Autodesk Fusion 360 part; units mm, degrees
note: some values were not read from the file. Set by a fixed rule: which sketch regions a step uses.
(part 11 of 20)
sketch "スケッチ2 (2)" plane through (0, 0, 8) normal (0, 0, 1) x (-1, 0, 0)
  circle A0 centre (-7.0711, -7.0711) radius 1.7
  circle A1 centre (7.0711, 7.0711) radius 1.7
  circle A2 centre (0, 10) radius 1.7
  circle A3 centre (0, -10) radius 1.7
  circle A4 centre (-10, 0) radius 1.7
  circle A5 centre (10, 0) radius 1.7
  circle A6 centre (-7.0711, 7.0711) radius 1.7
  circle A7 centre (7.0711, -7.0711) radius 1.7
  arc A8 (-13.5924, 2.0756) -> (-13.727, 0.7957) centre (0, 0) ccw
  line L0 (-13.727, 0.7957) -> (-14.4979, 0.8404)
  line L1 (-14.4979, 0.8404) -> (-14.4985, 0.8405)
  spline S0 degree 5 poles (-14.4985, 0.8405) (-14.4986, 0.8405) (-14.4987, 0.8405) (-14.499, 0.8405) (-14.4993, 0.8405) (-14.4999, 0.8405) (-14.5005, 0.8406) (-14.5012, 0.8406) (-14.502, 0.8406) (-14.5028, 0.8406) (-14.5037, 0.8407) (-14.5048, 0.8407) (-14.5058, 0.8407) (-14.507, 0.8407) (-14.5082, 0.8408) (-14.5096, 0.8408) (-14.5109, 0.8408) (-14.5124, 0.8408) (-14.5139, 0.8409) (-14.5155, 0.8409) (-14.5172, 0.8409) (-14.519, 0.8409) (-14.5208, 0.8409) (-14.5226, 0.8409) (-14.5246, 0.8409) (-14.5266, 0.8409) (-14.5287, 0.8409) (-14.5309, 0.8409) (-14.5331, 0.8408) (-14.5354, 0.8408) (-14.5377, 0.8408) (-14.5401, 0.8407) (-14.5426, 0.8407) (-14.5452, 0.8406) (-14.5478, 0.8406) (-14.5504, 0.8405) (-14.5532, 0.8404) (-14.556, 0.8403) (-14.5588, 0.8402) (-14.5617, 0.8401) (-14.5647, 0.84) (-14.5677, 0.8399) (-14.5708, 0.8398) (-14.574, 0.8396) (-14.5772, 0.8395) (-14.5805, 0.8393) (-14.5838, 0.8392) (-14.5872, 0.839) (-14.5906, 0.8388) (-14.5941, 0.8386) (-14.5977, 0.8384) (-14.6013, 0.8382) (-14.605, 0.838) (-14.6087, 0.8377) (-14.6124, 0.8375) (-14.6163, 0.8372) (-14.6202, 0.8369) (-14.6241, 0.8366) (-14.6281, 0.8363) (-14.6321, 0.836) (-14.6362, 0.8357) (-14.6404, 0.8354) (-14.6446, 0.835) (-14.6488, 0.8347) (-14.6531, 0.8343) (-14.6574, 0.8339) (-14.6618, 0.8335) (-14.6663, 0.8331) (-14.6708, 0.8326) (-14.6753, 0.8322) (-14.6799, 0.8317) (-14.6846, 0.8313) (-14.6893, 0.8308) (-14.694, 0.8303) (-14.6988, 0.8298) (-14.7036, 0.8292) (-14.7085, 0.8287) (-14.7134, 0.8281) (-14.7184, 0.8275) (-14.7234, 0.8269) (-14.7285, 0.8263) (-14.7336, 0.8257) (-14.7387, 0.8251) (-14.7439, 0.8244) (-14.7492, 0.8237) (-14.7545, 0.8231) (-14.7598, 0.8224) (-14.7652, 0.8216) (-14.7706, 0.8209) (-14.7761, 0.8201) (-14.7816, 0.8194) (-14.7871, 0.8186) (-14.7927, 0.8178) (-14.7983, 0.817) (-14.804, 0.8161) (-14.8097, 0.8153) (-14.8155, 0.8144) (-14.8213, 0.8135) (-14.8271, 0.8126) (-14.833, 0.8117) (-14.8389, 0.8107) (-14.8449, 0.8097) (-14.8509, 0.8088) (-14.8569, 0.8078) (-14.863, 0.8067) (-14.8691, 0.8057) (-14.8753, 0.8047) (-14.8814, 0.8036) (-14.8877, 0.8025) (-14.8939, 0.8014) (-14.9003, 0.8002) (-14.9066, 0.7991) (-14.913, 0.7979) (-14.9194, 0.7967) (-14.9259, 0.7955) (-14.9324, 0.7943) (-14.9389, 0.7931) (-14.9455, 0.7918) (-14.9521, 0.7905) (-14.9587, 0.7892) (-14.9654, 0.7879) (-14.9721, 0.7865) (-14.9788, 0.7852) (-14.9856, 0.7838) (-14.9924, 0.7824) (-14.9993, 0.781) (-15.0062, 0.7795) (-15.0131, 0.778) (-15.02, 0.7766) (-15.027, 0.775) (-15.0341, 0.7735) (-15.0411, 0.772) (-15.0482, 0.7704) (-15.0553, 0.7688) (-15.0625, 0.7672) (-15.0697, 0.7656) (-15.0769, 0.7639) (-15.0841, 0.7622) (-15.0914, 0.7605) (-15.0987, 0.7588) (-15.1061, 0.7571) (-15.1135, 0.7553) (-15.1209, 0.7535) (-15.1283, 0.7517) (-15.1358, 0.7499) (-15.1433, 0.7481) (-15.1508, 0.7462) (-15.1584, 0.7443) (-15.166, 0.7424) (-15.1736, 0.7405) (-15.1813, 0.7385) (-15.1889, 0.7365) (-15.1967, 0.7345) (-15.2044, 0.7325) (-15.2122, 0.7305) (-15.22, 0.7284) (-15.2278, 0.7263) (-15.2357, 0.7242) (-15.2436, 0.7221) (-15.2515, 0.7199) (-15.2594, 0.7177) (-15.2674, 0.7155) (-15.2754, 0.7133) (-15.2834, 0.7111) (-15.2915, 0.7088) (-15.2996, 0.7065) (-15.3077, 0.7042) (-15.3158, 0.7018) (-15.324, 0.6995) (-15.3322, 0.6971) (-15.3404, 0.6947) (-15.3487, 0.6923) (-15.3569, 0.6898) (-15.3652, 0.6873) (-15.3736, 0.6848) (-15.3819, 0.6823) (-15.3903, 0.6797) (-15.3987, 0.6772) (-15.4071, 0.6746) (-15.4156, 0.672) (-15.4241, 0.6693) (-15.4326, 0.6667) (-15.4411, 0.664) (-15.4497, 0.6613) (-15.4582, 0.6585) (-15.4668, 0.6558) (-15.4755, 0.653) (-15.4841, 0.6502) (-15.4928, 0.6473) (-15.5015, 0.6445) (-15.5102, 0.6416) (-15.519, 0.6387) (-15.5278, 0.6358) (-15.5365, 0.6328) (-15.5454, 0.6298) (-15.5542, 0.6268) (-15.5631, 0.6238) (-15.572, 0.6207) (-15.5809, 0.6177) (-15.5898, 0.6146) (-15.5988, 0.6114) (-15.6077, 0.6083) (-15.6167, 0.6051) (-15.6258, 0.6019) (-15.6348, 0.5987) (-15.6439, 0.5955) (-15.653, 0.5922) (-15.6621, 0.5889) (-15.6712, 0.5856) (-15.6803, 0.5822) (-15.6895, 0.5789) (-15.6987, 0.5755) (-15.7079, 0.572) (-15.7172, 0.5686) (-15.7264, 0.5651) (-15.7357, 0.5616) (-15.745, 0.5581) (-15.7543, 0.5546) (-15.7636, 0.551) (-15.773, 0.5474) (-15.7824, 0.5438) (-15.7918, 0.5401) (-15.8012, 0.5365) (-15.8106, 0.5328) (-15.8201, 0.529) (-15.8295, 0.5253) (-15.839, 0.5215) (-15.8486, 0.5177) (-15.8581, 0.5139) (-15.8676, 0.5101) (-15.8772, 0.5062) (-15.8868, 0.5023) (-15.8964, 0.4984) (-15.906, 0.4944) (-15.9157, 0.4904) (-15.9253, 0.4864) (-15.935, 0.4824) (-15.9447, 0.4784) (-15.9544, 0.4743) (-15.9641, 0.4702) (-15.9739, 0.466) (-15.9817, 0.4627) (-15.9876, 0.4602) (-15.9915, 0.4585) (-15.9935, 0.4577) knots 0 0 0 0 0 0 0.00416667 0.00833333 0.0125 0.01666667 0.02083333 0.025 0.02916667 0.03333333 0.0375 0.04166667 0.04583333 0.05 0.05416667 0.05833333 0.0625 0.06666667 0.07083333 0.075 0.07916667 0.08333333 0.0875 0.09166667 0.09583333 0.1 0.10416667 0.10833333 0.1125 0.11666667 0.12083333 0.125 0.12916667 0.13333333 0.1375 0.14166667 0.14583333 0.15 0.15416667 0.15833333 0.1625 0.16666667 0.17083333 0.175 0.17916667 0.18333333 0.1875 0.19166667 0.19583333 0.2 0.20416667 0.20833333 0.2125 0.21666667 0.22083333 0.225 0.22916667 0.23333333 0.2375 0.24166667 0.24583333 0.25 0.25416667 0.25833333 0.2625 0.26666667 0.27083333 0.275 0.27916667 0.28333333 0.2875 0.29166667 0.29583333 0.3 0.30416667 0.30833333 0.3125 0.31666667 0.32083333 0.325 0.32916667 0.33333333 0.3375 0.34166667 0.34583333 0.35 0.35416667 0.35833333 0.3625 0.36666667 0.37083333 0.375 0.37916667 0.38333333 0.3875 0.39166667 0.39583333 0.4 0.40416667 0.40833333 0.4125 0.41666667 0.42083333 0.425 0.42916667 0.43333333 0.4375 0.44166667 0.44583333 0.45 0.45416667 0.45833333 0.4625 0.46666667 0.47083333 0.475 0.47916667 0.48333333 0.4875 0.49166667 0.49583333 0.5 0.50416667 0.50833333 0.5125 0.51666667 0.52083333 0.525 0.52916667 0.53333333 0.5375 0.54166667 0.54583333 0.55 0.55416667 0.55833333 0.5625 0.56666667 0.57083333 0.575 0.57916667 0.58333333 0.5875 0.59166667 0.59583333 0.6 0.60416667 0.60833333 0.6125 0.61666667 0.62083333 0.625 0.62916667 0.63333333 0.6375 0.64166667 0.64583333 0.65 0.65416667 0.65833333 0.6625 0.66666667 0.67083333 0.675 0.67916667 0.68333333 0.6875 0.69166667 0.69583333 0.7 0.70416667 0.70833333 0.7125 0.71666667 0.72083333 0.725 0.72916667 0.73333333 0.7375 0.74166667 0.74583333 0.75 0.75416667 0.75833333 0.7625 0.76666667 0.77083333 0.775 0.77916667 0.78333333 0.7875 0.79166667 0.79583333 0.8 0.80416667 0.80833333 0.8125 0.81666667 0.82083333 0.825 0.82916667 0.83333333 0.8375 0.84166667 0.84583333 0.85 0.85416667 0.85833333 0.8625 0.86666667 0.87083333 0.875 0.87916667 0.88333333 0.8875 0.89166667 0.89583333 0.9 0.90416667 0.90833333 0.9125 0.91666667 0.92083333 0.925 0.92916667 0.93333333 0.9375 0.94166667 0.94583333 0.95 0.95416667 0.95833333 0.9625 0.96666667 0.97083333 0.975 0.97916667 0.98333333 0.9875 0.99166667 0.99583333 1 1 1 1 1 1
  arc A9 (-15.9935, 0.4577) -> (-15.9935, -0.4577) centre (0, 0) ccw
  spline S1 degree 5 poles (-15.9935, -0.4577) (-15.9915, -0.4585) (-15.9876, -0.4602) (-15.9817, -0.4627) (-15.9739, -0.466) (-15.9641, -0.4702) (-15.9544, -0.4743) (-15.9447, -0.4784) (-15.935, -0.4824) (-15.9253, -0.4864) (-15.9157, -0.4904) (-15.906, -0.4944) (-15.8964, -0.4984) (-15.8868, -0.5023) (-15.8772, -0.5062) (-15.8676, -0.5101) (-15.8581, -0.5139) (-15.8486, -0.5177) (-15.839, -0.5215) (-15.8295, -0.5253) (-15.8201, -0.529) (-15.8106, -0.5328) (-15.8012, -0.5365) (-15.7918, -0.5401) (-15.7824, -0.5438) (-15.773, -0.5474) (-15.7636, -0.551) (-15.7543, -0.5546) (-15.745, -0.5581) (-15.7357, -0.5616) (-15.7264, -0.5651) (-15.7172, -0.5686) (-15.7079, -0.572) (-15.6987, -0.5755) (-15.6895, -0.5789) (-15.6803, -0.5822) (-15.6712, -0.5856) (-15.6621, -0.5889) (-15.653, -0.5922) (-15.6439, -0.5955) (-15.6348, -0.5987) (-15.6258, -0.6019) (-15.6167, -0.6051) (-15.6077, -0.6083) (-15.5988, -0.6114) (-15.5898, -0.6146) (-15.5809, -0.6177) (-15.572, -0.6207) (-15.5631, -0.6238) (-15.5542, -0.6268) (-15.5454, -0.6298) (-15.5365, -0.6328) (-15.5278, -0.6358) (-15.519, -0.6387) (-15.5102, -0.6416) (-15.5015, -0.6445) (-15.4928, -0.6473) (-15.4841, -0.6502) (-15.4755, -0.653) (-15.4668, -0.6558) (-15.4582, -0.6585) (-15.4497, -0.6613) (-15.4411, -0.664) (-15.4326, -0.6667) (-15.4241, -0.6693) (-15.4156, -0.672) (-15.4071, -0.6746) (-15.3987, -0.6772) (-15.3903, -0.6797) (-15.3819, -0.6823) (-15.3736, -0.6848) (-15.3652, -0.6873) (-15.3569, -0.6898) (-15.3487, -0.6923) (-15.3404, -0.6947) (-15.3322, -0.6971) (-15.324, -0.6995) (-15.3158, -0.7018) (-15.3077, -0.7042) (-15.2996, -0.7065) (-15.2915, -0.7088) (-15.2834, -0.7111) (-15.2754, -0.7133) (-15.2674, -0.7155) (-15.2594, -0.7177) (-15.2515, -0.7199) (-15.2436, -0.7221) (-15.2357, -0.7242) (-15.2278, -0.7263) (-15.22, -0.7284) (-15.2122, -0.7305) (-15.2044, -0.7325) (-15.1967, -0.7345) (-15.1889, -0.7365) (-15.1813, -0.7385) (-15.1736, -0.7405) (-15.166, -0.7424) (-15.1584, -0.7443) (-15.1508, -0.7462) (-15.1433, -0.7481) (-15.1358, -0.7499) (-15.1283, -0.7517) (-15.1209, -0.7535) (-15.1135, -0.7553) (-15.1061, -0.7571) (-15.0987, -0.7588) (-15.0914, -0.7605) (-15.0841, -0.7622) (-15.0769, -0.7639) (-15.0697, -0.7656) (-15.0625, -0.7672) (-15.0553, -0.7688) (-15.0482, -0.7704) (-15.0411, -0.772) (-15.0341, -0.7735) (-15.027, -0.775) (-15.02, -0.7766) (-15.0131, -0.778) (-15.0062, -0.7795) (-14.9993, -0.781) (-14.9924, -0.7824) (-14.9856, -0.7838) (-14.9788, -0.7852) (-14.9721, -0.7865) (-14.9654, -0.7879) (-14.9587, -0.7892) (-14.9521, -0.7905) (-14.9455, -0.7918) (-14.9389, -0.7931) (-14.9324, -0.7943) (-14.9259, -0.7955) (-14.9194, -0.7967) (-14.913, -0.7979) (-14.9066, -0.7991) (-14.9003, -0.8002) (-14.8939, -0.8014) (-14.8877, -0.8025) (-14.8814, -0.8036) (-14.8753, -0.8047) (-14.8691, -0.8057) (-14.863, -0.8067) (-14.8569, -0.8078) (-14.8509, -0.8088) (-14.8449, -0.8097) (-14.8389, -0.8107) (-14.833, -0.8117) (-14.8271, -0.8126) (-14.8213, -0.8135) (-14.8155, -0.8144) (-14.8097, -0.8153) (-14.804, -0.8161) (-14.7983, -0.817) (-14.7927, -0.8178) (-14.7871, -0.8186) (-14.7816, -0.8194) (-14.7761, -0.8201) (-14.7706, -0.8209) (-14.7652, -0.8216) (-14.7598, -0.8224) (-14.7545, -0.8231) (-14.7492, -0.8237) (-14.7439, -0.8244) (-14.7387, -0.8251) (-14.7336, -0.8257) (-14.7285, -0.8263) (-14.7234, -0.8269) (-14.7184, -0.8275) (-14.7134, -0.8281) (-14.7085, -0.8287) (-14.7036, -0.8292) (-14.6988, -0.8298) (-14.694, -0.8303) (-14.6893, -0.8308) (-14.6846, -0.8313) (-14.6799, -0.8317) (-14.6753, -0.8322) (-14.6708, -0.8326) (-14.6663, -0.8331) (-14.6618, -0.8335) (-14.6574, -0.8339) (-14.6531, -0.8343) (-14.6488, -0.8347) (-14.6446, -0.835) (-14.6404, -0.8354) (-14.6362, -0.8357) (-14.6321, -0.836) (-14.6281, -0.8363) (-14.6241, -0.8366) (-14.6202, -0.8369) (-14.6163, -0.8372) (-14.6124, -0.8375) (-14.6087, -0.8377) (-14.605, -0.838) (-14.6013, -0.8382) (-14.5977, -0.8384) (-14.5941, -0.8386) (-14.5906, -0.8388) (-14.5872, -0.839) (-14.5838, -0.8392) (-14.5805, -0.8393) (-14.5772, -0.8395) (-14.574, -0.8396) (-14.5708, -0.8398) (-14.5677, -0.8399) (-14.5647, -0.84) (-14.5617, -0.8401) (-14.5588, -0.8402) (-14.556, -0.8403) (-14.5532, -0.8404) (-14.5504, -0.8405) (-14.5478, -0.8406) (-14.5452, -0.8406) (-14.5426, -0.8407) (-14.5401, -0.8407) (-14.5377, -0.8408) (-14.5354, -0.8408) (-14.5331, -0.8408) (-14.5309, -0.8409) (-14.5287, -0.8409) (-14.5266, -0.8409) (-14.5246, -0.8409) (-14.5226, -0.8409) (-14.5208, -0.8409) (-14.519, -0.8409) (-14.5172, -0.8409) (-14.5155, -0.8409) (-14.5139, -0.8409) (-14.5124, -0.8408) (-14.5109, -0.8408) (-14.5096, -0.8408) (-14.5082, -0.8408) (-14.507, -0.8407) (-14.5058, -0.8407) (-14.5048, -0.8407) (-14.5037, -0.8407) (-14.5028, -0.8406) (-14.502, -0.8406) (-14.5012, -0.8406) (-14.5005, -0.8406) (-14.4999, -0.8405) (-14.4993, -0.8405) (-14.499, -0.8405) (-14.4987, -0.8405) (-14.4986, -0.8405) (-14.4985, -0.8405) knots -1 -1 -1 -1 -1 -1 -0.99583333 -0.99166667 -0.9875 -0.98333333 -0.97916667 -0.975 -0.97083333 -0.96666667 -0.9625 -0.95833333 -0.95416667 -0.95 -0.94583333 -0.94166667 -0.9375 -0.93333333 -0.92916667 -0.925 -0.92083333 -0.91666667 -0.9125 -0.90833333 -0.90416667 -0.9 -0.89583333 -0.89166667 -0.8875 -0.88333333 -0.87916667 -0.875 -0.87083333 -0.86666667 -0.8625 -0.85833333 -0.85416667 -0.85 -0.84583333 -0.84166667 -0.8375 -0.83333333 -0.82916667 -0.825 -0.82083333 -0.81666667 -0.8125 -0.80833333 -0.80416667 -0.8 -0.79583333 -0.79166667 -0.7875 -0.78333333 -0.77916667 -0.775 -0.77083333 -0.76666667 -0.7625 -0.75833333 -0.75416667 -0.75 -0.74583333 -0.74166667 -0.7375 -0.73333333 -0.72916667 -0.725 -0.72083333 -0.71666667 -0.7125 -0.70833333 -0.70416667 -0.7 -0.69583333 -0.69166667 -0.6875 -0.68333333 -0.67916667 -0.675 -0.67083333 -0.66666667 -0.6625 -0.65833333 -0.65416667 -0.65 -0.64583333 -0.64166667 -0.6375 -0.63333333 -0.62916667 -0.625 -0.62083333 -0.61666667 -0.6125 -0.60833333 -0.60416667 -0.6 -0.59583333 -0.59166667 -0.5875 -0.58333333 -0.57916667 -0.575 -0.57083333 -0.56666667 -0.5625 -0.55833333 -0.55416667 -0.55 -0.54583333 -0.54166667 -0.5375 -0.53333333 -0.52916667 -0.525 -0.52083333 -0.51666667 -0.5125 -0.50833333 -0.50416667 -0.5 -0.49583333 -0.49166667 -0.4875 -0.48333333 -0.47916667 -0.475 -0.47083333 -0.46666667 -0.4625 -0.45833333 -0.45416667 -0.45 -0.44583333 -0.44166667 -0.4375 -0.43333333 -0.42916667 -0.425 -0.42083333 -0.41666667 -0.4125 -0.40833333 -0.40416667 -0.4 -0.39583333 -0.39166667 -0.3875 -0.38333333 -0.37916667 -0.375 -0.37083333 -0.36666667 -0.3625 -0.35833333 -0.35416667 -0.35 -0.34583333 -0.34166667 -0.3375 -0.33333333 -0.32916667 -0.325 -0.32083333 -0.31666667 -0.3125 -0.30833333 -0.30416667 -0.3 -0.29583333 -0.29166667 -0.2875 -0.28333333 -0.27916667 -0.275 -0.27083333 -0.26666667 -0.2625 -0.25833333 -0.25416667 -0.25 -0.24583333 -0.24166667 -0.2375 -0.23333333 -0.22916667 -0.225 -0.22083333 -0.21666667 -0.2125 -0.20833333 -0.20416667 -0.2 -0.19583333 -0.19166667 -0.1875 -0.18333333 -0.17916667 -0.175 -0.17083333 -0.16666667 -0.1625 -0.15833333 -0.15416667 -0.15 -0.14583333 -0.14166667 -0.1375 -0.13333333 -0.12916667 -0.125 -0.12083333 -0.11666667 -0.1125 -0.10833333 -0.10416667 -0.1 -0.09583333 -0.09166667 -0.0875 -0.08333333 -0.07916667 -0.075 -0.07083333 -0.06666667 -0.0625 -0.05833333 -0.05416667 -0.05 -0.04583333 -0.04166667 -0.0375 -0.03333333 -0.02916667 -0.025 -0.02083333 -0.01666667 -0.0125 -0.00833333 -0.00416667 0 0 0 0 0 0
  line L2 (-14.4985, -0.8405) -> (-14.4979, -0.8404)
  line L3 (-14.4979, -0.8404) -> (-13.727, -0.7957)
  arc A10 (-13.727, -0.7957) -> (-13.5924, -2.0756) centre (0, 0) ccw
  line L4 (-13.5924, -2.0756) -> (-14.3558, -2.1922)
  line L5 (-14.3558, -2.1922) -> (-14.3564, -2.1923)
  spline S2 degree 5 poles (-14.3564, -2.1923) (-14.3565, -2.1923) (-14.3566, -2.1923) (-14.3569, -2.1924) (-14.3572, -2.1924) (-14.3578, -2.1925) (-14.3584, -2.1926) (-14.3591, -2.1928) (-14.3598, -2.1929) (-14.3607, -2.193) (-14.3616, -2.1932) (-14.3626, -2.1934) (-14.3637, -2.1936) (-14.3648, -2.1938) (-14.366, -2.194) (-14.3673, -2.1943) (-14.3687, -2.1945) (-14.3701, -2.1948) (-14.3716, -2.1951) (-14.3732, -2.1954) (-14.3748, -2.1958) (-14.3765, -2.1961) (-14.3783, -2.1965) (-14.3801, -2.1969) (-14.382, -2.1973) (-14.384, -2.1977) (-14.386, -2.1982) (-14.3882, -2.1986) (-14.3903, -2.1991) (-14.3925, -2.1996) (-14.3948, -2.2002) (-14.3972, -2.2007) (-14.3996, -2.2013) (-14.4021, -2.2018) (-14.4046, -2.2025) (-14.4072, -2.2031) (-14.4099, -2.2037) (-14.4126, -2.2044) (-14.4154, -2.2051) (-14.4182, -2.2058) (-14.4211, -2.2065) (-14.424, -2.2072) (-14.427, -2.208) (-14.4301, -2.2088) (-14.4332, -2.2096) (-14.4364, -2.2104) (-14.4396, -2.2113) (-14.4429, -2.2122) (-14.4462, -2.2131) (-14.4496, -2.214) (-14.453, -2.2149) (-14.4565, -2.2159) (-14.46, -2.2169) (-14.4636, -2.2179) (-14.4673, -2.2189) (-14.4709, -2.22) (-14.4747, -2.2211) (-14.4785, -2.2222) (-14.4823, -2.2233) (-14.4862, -2.2244) (-14.4901, -2.2256) (-14.4941, -2.2268) (-14.4981, -2.228) (-14.5022, -2.2292) (-14.5063, -2.2305) (-14.5105, -2.2318) (-14.5147, -2.2331) (-14.519, -2.2344) (-14.5233, -2.2358) (-14.5277, -2.2372) (-14.5321, -2.2386) (-14.5365, -2.24) (-14.541, -2.2414) (-14.5455, -2.2429) (-14.5501, -2.2444) (-14.5547, -2.2459) (-14.5594, -2.2475) (-14.5641, -2.2491) (-14.5688, -2.2507) (-14.5736, -2.2523) (-14.5784, -2.2539) (-14.5833, -2.2556) (-14.5882, -2.2573) (-14.5932, -2.259) (-14.5981, -2.2608) (-14.6032, -2.2626) (-14.6082, -2.2644) (-14.6133, -2.2662) (-14.6185, -2.268) (-14.6237, -2.2699) (-14.6289, -2.2718) (-14.6342, -2.2737) (-14.6395, -2.2757) (-14.6448, -2.2776) (-14.6502, -2.2796) (-14.6556, -2.2817) (-14.661, -2.2837) (-14.6665, -2.2858) (-14.672, -2.2879) (-14.6776, -2.29) (-14.6832, -2.2922) (-14.6888, -2.2944) (-14.6945, -2.2966) (-14.7002, -2.2988) (-14.7059, -2.3011) (-14.7117, -2.3034) (-14.7175, -2.3057) (-14.7233, -2.308) (-14.7292, -2.3104) (-14.7351, -2.3128) (-14.741, -2.3152) (-14.747, -2.3176) (-14.753, -2.3201) (-14.759, -2.3226) (-14.7651, -2.3251) (-14.7712, -2.3277) (-14.7773, -2.3302) (-14.7835, -2.3328) (-14.7897, -2.3355) (-14.7959, -2.3381) (-14.8022, -2.3408) (-14.8084, -2.3435) (-14.8148, -2.3463) (-14.8211, -2.349) (-14.8275, -2.3518) (-14.8339, -2.3546) (-14.8403, -2.3575) (-14.8468, -2.3604) (-14.8533, -2.3633) (-14.8598, -2.3662) (-14.8663, -2.3691) (-14.8729, -2.3721) (-14.8795, -2.3751) (-14.8862, -2.3782) (-14.8928, -2.3812) (-14.8995, -2.3843) (-14.9062, -2.3874) (-14.913, -2.3906) (-14.9198, -2.3938) (-14.9266, -2.397) (-14.9334, -2.4002) (-14.9402, -2.4034) (-14.9471, -2.4067) (-14.954, -2.41) (-14.9609, -2.4134) (-14.9679, -2.4167) (-14.9749, -2.4201) (-14.9819, -2.4236) (-14.9889, -2.427) (-14.996, -2.4305) (-15.0031, -2.434) (-15.0102, -2.4375) (-15.0173, -2.4411) (-15.0245, -2.4447) (-15.0316, -2.4483) (-15.0388, -2.4519) (-15.0461, -2.4556) (-15.0533, -2.4593) (-15.0606, -2.463) (-15.0679, -2.4668) (-15.0752, -2.4706) (-15.0825, -2.4744) (-15.0899, -2.4782) (-15.0973, -2.4821) (-15.1047, -2.486) (-15.1121, -2.4899) (-15.1196, -2.4939) (-15.1271, -2.4978) (-15.1346, -2.5018) (-15.1421, -2.5059) (-15.1496, -2.5099) (-15.1572, -2.514) (-15.1648, -2.5182) (-15.1724, -2.5223) (-15.18, -2.5265) (-15.1876, -2.5307) (-15.1953, -2.5349) (-15.203, -2.5392) (-15.2107, -2.5435) (-15.2184, -2.5478) (-15.2262, -2.5522) (-15.2339, -2.5565) (-15.2417, -2.5609) (-15.2495, -2.5654) (-15.2574, -2.5698) (-15.2652, -2.5743) (-15.2731, -2.5788) (-15.2809, -2.5834) (-15.2888, -2.588) (-15.2968, -2.5926) (-15.3047, -2.5972) (-15.3126, -2.6019) (-15.3206, -2.6065) (-15.3286, -2.6113) (-15.3366, -2.616) (-15.3446, -2.6208) (-15.3527, -2.6256) (-15.3607, -2.6304) (-15.3688, -2.6353) (-15.3769, -2.6402) (-15.385, -2.6451) (-15.3931, -2.65) (-15.4013, -2.655) (-15.4094, -2.66) (-15.4176, -2.665) (-15.4258, -2.6701) (-15.434, -2.6752) (-15.4422, -2.6803) (-15.4505, -2.6855) (-15.4587, -2.6906) (-15.467, -2.6958) (-15.4753, -2.7011) (-15.4836, -2.7063) (-15.4919, -2.7116) (-15.5002, -2.7169) (-15.5086, -2.7223) (-15.517, -2.7277) (-15.5253, -2.7331) (-15.5337, -2.7385) (-15.5421, -2.744) (-15.5505, -2.7494) (-15.559, -2.755) (-15.5674, -2.7605) (-15.5759, -2.7661) (-15.5844, -2.7717) (-15.5929, -2.7773) (-15.6014, -2.783) (-15.6099, -2.7887) (-15.6184, -2.7944) (-15.6269, -2.8002) (-15.6355, -2.8059) (-15.6441, -2.8117) (-15.6526, -2.8176) (-15.6612, -2.8234) (-15.6698, -2.8293) (-15.6785, -2.8353) (-15.6871, -2.8412) (-15.6957, -2.8472) (-15.7044, -2.8532) (-15.713, -2.8592) (-15.7217, -2.8653) (-15.7287, -2.8702) (-15.7339, -2.8738) (-15.7374, -2.8763) (-15.7391, -2.8775) knots 0 0 0 0 0 0 0.00416667 0.00833333 0.0125 0.01666667 0.02083333 0.025 0.02916667 0.03333333 0.0375 0.04166667 0.04583333 0.05 0.05416667 0.05833333 0.0625 0.06666667 0.07083333 0.075 0.07916667 0.08333333 0.0875 0.09166667 0.09583333 0.1 0.10416667 0.10833333 0.1125 0.11666667 0.12083333 0.125 0.12916667 0.13333333 0.1375 0.14166667 0.14583333 0.15 0.15416667 0.15833333 0.1625 0.16666667 0.17083333 0.175 0.17916667 0.18333333 0.1875 0.19166667 0.19583333 0.2 0.20416667 0.20833333 0.2125 0.21666667 0.22083333 0.225 0.22916667 0.23333333 0.2375 0.24166667 0.24583333 0.25 0.25416667 0.25833333 0.2625 0.26666667 0.27083333 0.275 0.27916667 0.28333333 0.2875 0.29166667 0.29583333 0.3 0.30416667 0.30833333 0.3125 0.31666667 0.32083333 0.325 0.32916667 0.33333333 0.3375 0.34166667 0.34583333 0.35 0.35416667 0.35833333 0.3625 0.36666667 0.37083333 0.375 0.37916667 0.38333333 0.3875 0.39166667 0.39583333 0.4 0.40416667 0.40833333 0.4125 0.41666667 0.42083333 0.425 0.42916667 0.43333333 0.4375 0.44166667 0.44583333 0.45 0.45416667 0.45833333 0.4625 0.46666667 0.47083333 0.475 0.47916667 0.48333333 0.4875 0.49166667 0.49583333 0.5 0.50416667 0.50833333 0.5125 0.51666667 0.52083333 0.525 0.52916667 0.53333333 0.5375 0.54166667 0.54583333 0.55 0.55416667 0.55833333 0.5625 0.56666667 0.57083333 0.575 0.57916667 0.58333333 0.5875 0.59166667 0.59583333 0.6 0.60416667 0.60833333 0.6125 0.61666667 0.62083333 0.625 0.62916667 0.63333333 0.6375 0.64166667 0.64583333 0.65 0.65416667 0.65833333 0.6625 0.66666667 0.67083333 0.675 0.67916667 0.68333333 0.6875 0.69166667 0.69583333 0.7 0.70416667 0.70833333 0.7125 0.71666667 0.72083333 0.725 0.72916667 0.73333333 0.7375 0.74166667 0.74583333 0.75 0.75416667 0.75833333 0.7625 0.76666667 0.77083333 0.775 0.77916667 0.78333333 0.7875 0.79166667 0.79583333 0.8 0.80416667 0.80833333 0.8125 0.81666667 0.82083333 0.825 0.82916667 0.83333333 0.8375 0.84166667 0.84583333 0.85 0.85416667 0.85833333 0.8625 0.86666667 0.87083333 0.875 0.87916667 0.88333333 0.8875 0.89166667 0.89583333 0.9 0.90416667 0.90833333 0.9125 0.91666667 0.92083333 0.925 0.92916667 0.93333333 0.9375 0.94166667 0.94583333 0.95 0.95416667 0.95833333 0.9625 0.96666667 0.97083333 0.975 0.97916667 0.98333333 0.9875 0.99166667 0.99583333 1 1 1 1 1 1
  arc A11 (-15.7391, -2.8775) -> (-15.5488, -3.7729) centre (0, 0) ccw
  spline S3 degree 5 poles (-15.5488, -3.7729) (-15.5467, -3.7733) (-15.5425, -3.7742) (-15.5363, -3.7754) (-15.5279, -3.777) (-15.5175, -3.779) (-15.5072, -3.781) (-15.4968, -3.783) (-15.4865, -3.7849) (-15.4762, -3.7869) (-15.4659, -3.7888) (-15.4556, -3.7907) (-15.4454, -3.7925) (-15.4352, -3.7944) (-15.425, -3.7962) (-15.4148, -3.798) (-15.4047, -3.7998) (-15.3946, -3.8015) (-15.3845, -3.8033) (-15.3744, -3.805) (-15.3644, -3.8067) (-15.3544, -3.8083) (-15.3444, -3.81) (-15.3344, -3.8116) (-15.3244, -3.8132) (-15.3145, -3.8148) (-15.3046, -3.8164) (-15.2947, -3.8179) (-15.2849, -3.8195) (-15.2751, -3.821) (-15.2653, -3.8225) (-15.2555, -3.8239) (-15.2457, -3.8254) (-15.236, -3.8268) (-15.2263, -3.8282) (-15.2166, -3.8296) (-15.207, -3.831) (-15.1974, -3.8323) (-15.1878, -3.8337) (-15.1782, -3.835) (-15.1687, -3.8363) (-15.1591, -3.8375) (-15.1497, -3.8388) (-15.1402, -3.84) (-15.1308, -3.8412) (-15.1214, -3.8424) (-15.112, -3.8436) (-15.1026, -3.8448) (-15.0933, -3.8459) (-15.084, -3.847) (-15.0747, -3.8481) (-15.0655, -3.8492) (-15.0563, -3.8503) (-15.0471, -3.8513) (-15.0379, -3.8523) (-15.0288, -3.8533) (-15.0197, -3.8543) (-15.0106, -3.8553) (-15.0015, -3.8562) (-14.9925, -3.8572) (-14.9835, -3.8581) (-14.9746, -3.859) (-14.9656, -3.8598) (-14.9567, -3.8607) (-14.9479, -3.8615) (-14.939, -3.8624) (-14.9302, -3.8632) (-14.9214, -3.8639) (-14.9127, -3.8647) (-14.9039, -3.8655) (-14.8952, -3.8662) (-14.8866, -3.8669) (-14.8779, -3.8676) (-14.8693, -3.8683) (-14.8608, -3.869) (-14.8522, -3.8696) (-14.8437, -3.8702) (-14.8352, -3.8708) (-14.8268, -3.8714) (-14.8184, -3.872) (-14.81, -3.8726) (-14.8016, -3.8731) (-14.7933, -3.8737) (-14.785, -3.8742) (-14.7768, -3.8747) (-14.7685, -3.8751) (-14.7603, -3.8756) (-14.7522, -3.8761) (-14.744, -3.8765) (-14.7359, -3.8769) (-14.7279, -3.8773) (-14.7199, -3.8777) (-14.7119, -3.878) (-14.7039, -3.8784) (-14.696, -3.8787) (-14.6881, -3.8791) (-14.6802, -3.8794) (-14.6724, -3.8797) (-14.6646, -3.8799) (-14.6568, -3.8802) (-14.6491, -3.8804) (-14.6414, -3.8807) (-14.6338, -3.8809) (-14.6261, -3.8811) (-14.6186, -3.8813) (-14.611, -3.8814) (-14.6035, -3.8816) (-14.596, -3.8817) (-14.5886, -3.8819) (-14.5812, -3.882) (-14.5738, -3.8821) (-14.5665, -3.8822) (-14.5592, -3.8823) (-14.5519, -3.8823) (-14.5447, -3.8824) (-14.5375, -3.8824) (-14.5304, -3.8824) (-14.5233, -3.8824) (-14.5162, -3.8824) (-14.5091, -3.8824) (-14.5021, -3.8824) (-14.4952, -3.8823) (-14.4883, -3.8823) (-14.4814, -3.8822) (-14.4745, -3.8821) (-14.4677, -3.882) (-14.461, -3.8819) (-14.4542, -3.8818) (-14.4476, -3.8817) (-14.4409, -3.8816) (-14.4343, -3.8814) (-14.4277, -3.8812) (-14.4212, -3.8811) (-14.4147, -3.8809) (-14.4083, -3.8807) (-14.4019, -3.8805) (-14.3955, -3.8803) (-14.3892, -3.88) (-14.3829, -3.8798) (-14.3767, -3.8796) (-14.3705, -3.8793) (-14.3643, -3.879) (-14.3582, -3.8788) (-14.3521, -3.8785) (-14.3461, -3.8782) (-14.3401, -3.8779) (-14.3342, -3.8776) (-14.3283, -3.8772) (-14.3224, -3.8769) (-14.3166, -3.8766) (-14.3108, -3.8762) (-14.3051, -3.8758) (-14.2994, -3.8755) (-14.2938, -3.8751) (-14.2882, -3.8747) (-14.2826, -3.8743) (-14.2771, -3.8739) (-14.2717, -3.8735) (-14.2663, -3.8731) (-14.2609, -3.8727) (-14.2556, -3.8723) (-14.2503, -3.8718) (-14.2451, -3.8714) (-14.2399, -3.871) (-14.2348, -3.8705) (-14.2297, -3.87) (-14.2247, -3.8696) (-14.2197, -3.8691) (-14.2148, -3.8686) (-14.2099, -3.8682) (-14.2051, -3.8677) (-14.2003, -3.8672) (-14.1955, -3.8667) (-14.1908, -3.8662) (-14.1862, -3.8657) (-14.1816, -3.8652) (-14.1771, -3.8647) (-14.1726, -3.8642) (-14.1682, -3.8636) (-14.1638, -3.8631) (-14.1594, -3.8626) (-14.1552, -3.8621) (-14.1509, -3.8615) (-14.1467, -3.861) (-14.1426, -3.8605) (-14.1386, -3.86) (-14.1345, -3.8594) (-14.1306, -3.8589) (-14.1267, -3.8583) (-14.1228, -3.8578) (-14.119, -3.8573) (-14.1153, -3.8567) (-14.1116, -3.8562) (-14.1079, -3.8557) (-14.1044, -3.8551) (-14.1009, -3.8546) (-14.0974, -3.854) (-14.094, -3.8535) (-14.0906, -3.853) (-14.0873, -3.8525) (-14.0841, -3.8519) (-14.0809, -3.8514) (-14.0778, -3.8509) (-14.0748, -3.8504) (-14.0718, -3.8498) (-14.0688, -3.8493) (-14.066, -3.8488) (-14.0632, -3.8483) (-14.0604, -3.8478) (-14.0577, -3.8473) (-14.0551, -3.8469) (-14.0525, -3.8464) (-14.05, -3.8459) (-14.0476, -3.8454) (-14.0452, -3.845) (-14.0429, -3.8445) (-14.0407, -3.8441) (-14.0385, -3.8436) (-14.0364, -3.8432) (-14.0343, -3.8428) (-14.0324, -3.8424) (-14.0305, -3.842) (-14.0286, -3.8416) (-14.0268, -3.8412) (-14.0251, -3.8408) (-14.0235, -3.8405) (-14.0219, -3.8401) (-14.0204, -3.8398) (-14.019, -3.8394) (-14.0177, -3.8391) (-14.0164, -3.8388) (-14.0152, -3.8386) (-14.0141, -3.8383) (-14.013, -3.838) (-14.012, -3.8378) (-14.0111, -3.8376) (-14.0103, -3.8374) (-14.0095, -3.8372) (-14.0089, -3.837) (-14.0083, -3.8369) (-14.0077, -3.8367) (-14.0074, -3.8366) (-14.0072, -3.8366) (-14.007, -3.8365) (-14.007, -3.8365) knots -1 -1 -1 -1 -1 -1 -0.99583333 -0.99166667 -0.9875 -0.98333333 -0.97916667 -0.975 -0.97083333 -0.96666667 -0.9625 -0.95833333 -0.95416667 -0.95 -0.94583333 -0.94166667 -0.9375 -0.93333333 -0.92916667 -0.925 -0.92083333 -0.91666667 -0.9125 -0.90833333 -0.90416667 -0.9 -0.89583333 -0.89166667 -0.8875 -0.88333333 -0.87916667 -0.875 -0.87083333 -0.86666667 -0.8625 -0.85833333 -0.85416667 -0.85 -0.84583333 -0.84166667 -0.8375 -0.83333333 -0.82916667 -0.825 -0.82083333 -0.81666667 -0.8125 -0.80833333 -0.80416667 -0.8 -0.79583333 -0.79166667 -0.7875 -0.78333333 -0.77916667 -0.775 -0.77083333 -0.76666667 -0.7625 -0.75833333 -0.75416667 -0.75 -0.74583333 -0.74166667 -0.7375 -0.73333333 -0.72916667 -0.725 -0.72083333 -0.71666667 -0.7125 -0.70833333 -0.70416667 -0.7 -0.69583333 -0.69166667 -0.6875 -0.68333333 -0.67916667 -0.675 -0.67083333 -0.66666667 -0.6625 -0.65833333 -0.65416667 -0.65 -0.64583333 -0.64166667 -0.6375 -0.63333333 -0.62916667 -0.625 -0.62083333 -0.61666667 -0.6125 -0.60833333 -0.60416667 -0.6 -0.59583333 -0.59166667 -0.5875 -0.58333333 -0.57916667 -0.575 -0.57083333 -0.56666667 -0.5625 -0.55833333 -0.55416667 -0.55 -0.54583333 -0.54166667 -0.5375 -0.53333333 -0.52916667 -0.525 -0.52083333 -0.51666667 -0.5125 -0.50833333 -0.50416667 -0.5 -0.49583333 -0.49166667 -0.4875 -0.48333333 -0.47916667 -0.475 -0.47083333 -0.46666667 -0.4625 -0.45833333 -0.45416667 -0.45 -0.44583333 -0.44166667 -0.4375 -0.43333333 -0.42916667 -0.425 -0.42083333 -0.41666667 -0.4125 -0.40833333 -0.40416667 -0.4 -0.39583333 -0.39166667 -0.3875 -0.38333333 -0.37916667 -0.375 -0.37083333 -0.36666667 -0.3625 -0.35833333 -0.35416667 -0.35 -0.34583333 -0.34166667 -0.3375 -0.33333333 -0.32916667 -0.325 -0.32083333 -0.31666667 -0.3125 -0.30833333 -0.30416667 -0.3 -0.29583333 -0.29166667 -0.2875 -0.28333333 -0.27916667 -0.275 -0.27083333 -0.26666667 -0.2625 -0.25833333 -0.25416667 -0.25 -0.24583333 -0.24166667 -0.2375 -0.23333333 -0.22916667 -0.225 -0.22083333 -0.21666667 -0.2125 -0.20833333 -0.20416667 -0.2 -0.19583333 -0.19166667 -0.1875 -0.18333333 -0.17916667 -0.175 -0.17083333 -0.16666667 -0.1625 -0.15833333 -0.15416667 -0.15 -0.14583333 -0.14166667 -0.1375 -0.13333333 -0.12916667 -0.125 -0.12083333 -0.11666667 -0.1125 -0.10833333 -0.10416667 -0.1 -0.09583333 -0.09166667 -0.0875 -0.08333333 -0.07916667 -0.075 -0.07083333 -0.06666667 -0.0625 -0.05833333 -0.05416667 -0.05 -0.04583333 -0.04166667 -0.0375 -0.03333333 -0.02916667 -0.025 -0.02083333 -0.01666667 -0.0125 -0.00833333 -0.00416667 0 0 0 0 0 0
  line L6 (-14.007, -3.8365) -> (-14.0063, -3.8363)
  line L7 (-14.0063, -3.8363) -> (-13.2615, -3.6324)
  arc A12 (-13.2615, -3.6324) -> (-12.8639, -4.8563) centre (0, 0) ccw
  line L8 (-12.8639, -4.8563) -> (-13.5863, -5.129)
  line L9 (-13.5863, -5.129) -> (-13.5869, -5.1293)
  spline S4 degree 5 poles (-13.5869, -5.1293) (-13.587, -5.1293) (-13.5871, -5.1293) (-13.5873, -5.1294) (-13.5877, -5.1296) (-13.5882, -5.1298) (-13.5887, -5.13) (-13.5894, -5.1303) (-13.5901, -5.1305) (-13.5909, -5.1309) (-13.5918, -5.1312) (-13.5927, -5.1316) (-13.5937, -5.132) (-13.5948, -5.1325) (-13.5959, -5.1329) (-13.5971, -5.1335) (-13.5984, -5.134) (-13.5997, -5.1346) (-13.6011, -5.1352) (-13.6026, -5.1358) (-13.6042, -5.1365) (-13.6057, -5.1372) (-13.6074, -5.1379) (-13.6091, -5.1387) (-13.6109, -5.1395) (-13.6128, -5.1403) (-13.6147, -5.1412) (-13.6166, -5.1421) (-13.6186, -5.143) (-13.6207, -5.1439) (-13.6228, -5.1449) (-13.625, -5.146) (-13.6273, -5.147) (-13.6296, -5.1481) (-13.6319, -5.1492) (-13.6343, -5.1504) (-13.6368, -5.1515) (-13.6393, -5.1528) (-13.6419, -5.154) (-13.6445, -5.1553) (-13.6472, -5.1566) (-13.6499, -5.1579) (-13.6527, -5.1593) (-13.6555, -5.1607) (-13.6584, -5.1622) (-13.6613, -5.1636) (-13.6643, -5.1651) (-13.6673, -5.1667) (-13.6704, -5.1682) (-13.6735, -5.1698) (-13.6767, -5.1715) (-13.6799, -5.1732) (-13.6831, -5.1749) (-13.6864, -5.1766) (-13.6898, -5.1783) (-13.6932, -5.1801) (-13.6966, -5.182) (-13.7001, -5.1838) (-13.7036, -5.1857) (-13.7072, -5.1877) (-13.7108, -5.1896) (-13.7144, -5.1916) (-13.7181, -5.1936) (-13.7218, -5.1957) (-13.7256, -5.1978) (-13.7294, -5.1999) (-13.7333, -5.2021) (-13.7372, -5.2043) (-13.7411, -5.2065) (-13.7451, -5.2087) (-13.7491, -5.211) (-13.7531, -5.2134) (-13.7572, -5.2157) (-13.7613, -5.2181) (-13.7655, -5.2205) (-13.7697, -5.223) (-13.7739, -5.2254) (-13.7782, -5.228) (-13.7825, -5.2305) (-13.7869, -5.2331) (-13.7912, -5.2357) (-13.7956, -5.2384) (-13.8001, -5.241) (-13.8046, -5.2438) (-13.8091, -5.2465) (-13.8136, -5.2493) (-13.8182, -5.2521) (-13.8228, -5.2549) (-13.8275, -5.2578) (-13.8322, -5.2607) (-13.8369, -5.2637) (-13.8416, -5.2666) (-13.8464, -5.2697) (-13.8512, -5.2727) (-13.8561, -5.2758) (-13.8609, -5.2789) (-13.8658, -5.282) (-13.8708, -5.2852) (-13.8757, -5.2884) (-13.8807, -5.2916) (-13.8858, -5.2949) (-13.8908, -5.2982) (-13.8959, -5.3015) (-13.901, -5.3049) (-13.9061, -5.3083) (-13.9113, -5.3118) (-13.9165, -5.3152) (-13.9217, -5.3187) (-13.927, -5.3223) (-13.9322, -5.3258) (-13.9376, -5.3294) (-13.9429, -5.3331) (-13.9482, -5.3367) (-13.9536, -5.3404) (-13.959, -5.3441) (-13.9645, -5.3479) (-13.9699, -5.3517) (-13.9754, -5.3555) (-13.9809, -5.3594) (-13.9865, -5.3633) (-13.992, -5.3672) (-13.9976, -5.3712) (-14.0032, -5.3752) (-14.0088, -5.3792) (-14.0145, -5.3832) (-14.0202, -5.3873) (-14.0259, -5.3914) (-14.0316, -5.3956) (-14.0373, -5.3998) (-14.0431, -5.404) (-14.0489, -5.4083) (-14.0547, -5.4125) (-14.0606, -5.4169) (-14.0664, -5.4212) (-14.0723, -5.4256) (-14.0782, -5.43) (-14.0841, -5.4344) (-14.0901, -5.4389) (-14.096, -5.4434) (-14.102, -5.448) (-14.108, -5.4526) (-14.114, -5.4572) (-14.1201, -5.4618) (-14.1262, -5.4665) (-14.1322, -5.4712) (-14.1383, -5.4759) (-14.1445, -5.4807) (-14.1506, -5.4855) (-14.1568, -5.4903) (-14.163, -5.4952) (-14.1692, -5.5001) (-14.1754, -5.505) (-14.1816, -5.51) (-14.1879, -5.515) (-14.1941, -5.52) (-14.2004, -5.5251) (-14.2067, -5.5302) (-14.213, -5.5353) (-14.2194, -5.5405) (-14.2257, -5.5457) (-14.2321, -5.5509) (-14.2385, -5.5561) (-14.2449, -5.5614) (-14.2513, -5.5667) (-14.2578, -5.5721) (-14.2642, -5.5775) (-14.2707, -5.5829) (-14.2772, -5.5883) (-14.2837, -5.5938) (-14.2902, -5.5993) (-14.2967, -5.6049) (-14.3033, -5.6105) (-14.3098, -5.6161) (-14.3164, -5.6217) (-14.323, -5.6274) (-14.3296, -5.6331) (-14.3362, -5.6388) (-14.3429, -5.6446) (-14.3495, -5.6504) (-14.3562, -5.6562) (-14.3628, -5.6621) (-14.3695, -5.668) (-14.3762, -5.6739) (-14.3829, -5.6799) (-14.3896, -5.6859) (-14.3964, -5.6919) (-14.4031, -5.6979) (-14.4099, -5.704) (-14.4167, -5.7101) (-14.4235, -5.7163) (-14.4303, -5.7225) (-14.4371, -5.7287) (-14.4439, -5.7349) (-14.4507, -5.7412) (-14.4576, -5.7475) (-14.4644, -5.7538) (-14.4713, -5.7602) (-14.4782, -5.7666) (-14.4851, -5.773) (-14.492, -5.7795) (-14.4989, -5.786) (-14.5058, -5.7925) (-14.5127, -5.7991) (-14.5197, -5.8057) (-14.5266, -5.8123) (-14.5336, -5.819) (-14.5405, -5.8256) (-14.5475, -5.8324) (-14.5545, -5.8391) (-14.5615, -5.8459) (-14.5685, -5.8527) (-14.5755, -5.8595) (-14.5826, -5.8664) (-14.5896, -5.8733) (-14.5966, -5.8802) (-14.6037, -5.8872) (-14.6108, -5.8942) (-14.6178, -5.9012) (-14.6249, -5.9083) (-14.632, -5.9154) (-14.6391, -5.9225) (-14.6462, -5.9297) (-14.6533, -5.9368) (-14.6604, -5.9441) (-14.6675, -5.9513) (-14.6747, -5.9586) (-14.6818, -5.9659) (-14.689, -5.9732) (-14.6961, -5.9806) (-14.7033, -5.988) (-14.7104, -5.9954) (-14.7176, -6.0029) (-14.7248, -6.0104) (-14.732, -6.0179) (-14.7392, -6.0254) (-14.7464, -6.033) (-14.7536, -6.0406) (-14.7608, -6.0483) (-14.768, -6.056) (-14.7752, -6.0637) (-14.7824, -6.0714) (-14.7882, -6.0776) (-14.7926, -6.0823) (-14.7955, -6.0854) (-14.7969, -6.087) knots 0 0 0 0 0 0 0.00416667 0.00833333 0.0125 0.01666667 0.02083333 0.025 0.02916667 0.03333333 0.0375 0.04166667 0.04583333 0.05 0.05416667 0.05833333 0.0625 0.06666667 0.07083333 0.075 0.07916667 0.08333333 0.0875 0.09166667 0.09583333 0.1 0.10416667 0.10833333 0.1125 0.11666667 0.12083333 0.125 0.12916667 0.13333333 0.1375 0.14166667 0.14583333 0.15 0.15416667 0.15833333 0.1625 0.16666667 0.17083333 0.175 0.17916667 0.18333333 0.1875 0.19166667 0.19583333 0.2 0.20416667 0.20833333 0.2125 0.21666667 0.22083333 0.225 0.22916667 0.23333333 0.2375 0.24166667 0.24583333 0.25 0.25416667 0.25833333 0.2625 0.26666667 0.27083333 0.275 0.27916667 0.28333333 0.2875 0.29166667 0.29583333 0.3 0.30416667 0.30833333 0.3125 0.31666667 0.32083333 0.325 0.32916667 0.33333333 0.3375 0.34166667 0.34583333 0.35 0.35416667 0.35833333 0.3625 0.36666667 0.37083333 0.375 0.37916667 0.38333333 0.3875 0.39166667 0.39583333 0.4 0.40416667 0.40833333 0.4125 0.41666667 0.42083333 0.425 0.42916667 0.43333333 0.4375 0.44166667 0.44583333 0.45 0.45416667 0.45833333 0.4625 0.46666667 0.47083333 0.475 0.47916667 0.48333333 0.4875 0.49166667 0.49583333 0.5 0.50416667 0.50833333 0.5125 0.51666667 0.52083333 0.525 0.52916667 0.53333333 0.5375 0.54166667 0.54583333 0.55 0.55416667 0.55833333 0.5625 0.56666667 0.57083333 0.575 0.57916667 0.58333333 0.5875 0.59166667 0.59583333 0.6 0.60416667 0.60833333 0.6125 0.61666667 0.62083333 0.625 0.62916667 0.63333333 0.6375 0.64166667 0.64583333 0.65 0.65416667 0.65833333 0.6625 0.66666667 0.67083333 0.675 0.67916667 0.68333333 0.6875 0.69166667 0.69583333 0.7 0.70416667 0.70833333 0.7125 0.71666667 0.72083333 0.725 0.72916667 0.73333333 0.7375 0.74166667 0.74583333 0.75 0.75416667 0.75833333 0.7625 0.76666667 0.77083333 0.775 0.77916667 0.78333333 0.7875 0.79166667 0.79583333 0.8 0.80416667 0.80833333 0.8125 0.81666667 0.82083333 0.825 0.82916667 0.83333333 0.8375 0.84166667 0.84583333 0.85 0.85416667 0.85833333 0.8625 0.86666667 0.87083333 0.875 0.87916667 0.88333333 0.8875 0.89166667 0.89583333 0.9 0.90416667 0.90833333 0.9125 0.91666667 0.92083333 0.925 0.92916667 0.93333333 0.9375 0.94166667 0.94583333 0.95 0.95416667 0.95833333 0.9625 0.96666667 0.97083333 0.975 0.97916667 0.98333333 0.9875 0.99166667 0.99583333 1 1 1 1 1 1
  arc A13 (-14.7969, -6.087) -> (-14.4246, -6.9233) centre (0, 0) ccw
  spline S5 degree 5 poles (-14.4246, -6.9233) (-14.4224, -6.9232) (-14.4182, -6.9232) (-14.4118, -6.9231) (-14.4033, -6.9229) (-14.3927, -6.9227) (-14.3822, -6.9225) (-14.3716, -6.9223) (-14.3611, -6.9221) (-14.3507, -6.9218) (-14.3402, -6.9215) (-14.3298, -6.9212) (-14.3194, -6.9209) (-14.309, -6.9206) (-14.2987, -6.9203) (-14.2883, -6.9199) (-14.2781, -6.9195) (-14.2678, -6.9192) (-14.2576, -6.9188) (-14.2474, -6.9183) (-14.2372, -6.9179) (-14.227, -6.9175) (-14.2169, -6.917) (-14.2068, -6.9165) (-14.1967, -6.916) (-14.1867, -6.9155) (-14.1767, -6.915) (-14.1667, -6.9145) (-14.1568, -6.9139) (-14.1468, -6.9134) (-14.1369, -6.9128) (-14.1271, -6.9122) (-14.1172, -6.9116) (-14.1074, -6.9109) (-14.0976, -6.9103) (-14.0879, -6.9097) (-14.0782, -6.909) (-14.0685, -6.9083) (-14.0588, -6.9076) (-14.0492, -6.9069) (-14.0396, -6.9062) (-14.03, -6.9055) (-14.0205, -6.9047) (-14.011, -6.9039) (-14.0015, -6.9032) (-13.992, -6.9024) (-13.9826, -6.9016) (-13.9732, -6.9008) (-13.9639, -6.8999) (-13.9545, -6.8991) (-13.9452, -6.8982) (-13.936, -6.8974) (-13.9267, -6.8965) (-13.9175, -6.8956) (-13.9083, -6.8947) (-13.8992, -6.8938) (-13.8901, -6.8929) (-13.881, -6.8919) (-13.872, -6.891) (-13.8629, -6.89) (-13.854, -6.889) (-13.845, -6.888) (-13.8361, -6.887) (-13.8272, -6.886) (-13.8184, -6.885) (-13.8095, -6.884) (-13.8007, -6.8829) (-13.792, -6.8818) (-13.7833, -6.8808) (-13.7746, -6.8797) (-13.7659, -6.8786) (-13.7573, -6.8775) (-13.7487, -6.8764) (-13.7401, -6.8753) (-13.7316, -6.8741) (-13.7231, -6.873) (-13.7147, -6.8718) (-13.7063, -6.8707) (-13.6979, -6.8695) (-13.6895, -6.8683) (-13.6812, -6.8671) (-13.6729, -6.8659) (-13.6647, -6.8647) (-13.6564, -6.8635) (-13.6483, -6.8623) (-13.6401, -6.861) (-13.632, -6.8598) (-13.6239, -6.8585) (-13.6159, -6.8572) (-13.6079, -6.856) (-13.5999, -6.8547) (-13.592, -6.8534) (-13.5841, -6.8521) (-13.5762, -6.8508) (-13.5684, -6.8494) (-13.5606, -6.8481) (-13.5528, -6.8468) (-13.5451, -6.8454) (-13.5375, -6.8441) (-13.5298, -6.8427) (-13.5222, -6.8414) (-13.5146, -6.84) (-13.5071, -6.8386) (-13.4996, -6.8372) (-13.4922, -6.8358) (-13.4847, -6.8344) (-13.4773, -6.833) (-13.47, -6.8316) (-13.4627, -6.8302) (-13.4554, -6.8288) (-13.4482, -6.8273) (-13.441, -6.8259) (-13.4339, -6.8244) (-13.4267, -6.823) (-13.4197, -6.8215) (-13.4126, -6.8201) (-13.4056, -6.8186) (-13.3987, -6.8171) (-13.3918, -6.8157) (-13.3849, -6.8142) (-13.378, -6.8127) (-13.3712, -6.8112) (-13.3645, -6.8097) (-13.3578, -6.8082) (-13.3511, -6.8067) (-13.3445, -6.8052) (-13.3379, -6.8037) (-13.3313, -6.8022) (-13.3248, -6.8007) (-13.3183, -6.7992) (-13.3119, -6.7976) (-13.3055, -6.7961) (-13.2991, -6.7946) (-13.2928, -6.7931) (-13.2866, -6.7915) (-13.2804, -6.79) (-13.2742, -6.7885) (-13.268, -6.7869) (-13.2619, -6.7854) (-13.2559, -6.7839) (-13.2499, -6.7823) (-13.2439, -6.7808) (-13.238, -6.7792) (-13.2321, -6.7777) (-13.2263, -6.7761) (-13.2205, -6.7746) (-13.2147, -6.7731) (-13.209, -6.7715) (-13.2034, -6.77) (-13.1978, -6.7684) (-13.1922, -6.7669) (-13.1867, -6.7653) (-13.1812, -6.7638) (-13.1758, -6.7623) (-13.1704, -6.7607) (-13.165, -6.7592) (-13.1597, -6.7577) (-13.1545, -6.7561) (-13.1493, -6.7546) (-13.1441, -6.7531) (-13.139, -6.7516) (-13.1339, -6.75) (-13.1289, -6.7485) (-13.124, -6.747) (-13.119, -6.7455) (-13.1142, -6.744) (-13.1093, -6.7425) (-13.1046, -6.741) (-13.0998, -6.7395) (-13.0951, -6.738) (-13.0905, -6.7366) (-13.0859, -6.7351) (-13.0814, -6.7336) (-13.0769, -6.7321) (-13.0725, -6.7307) (-13.0681, -6.7292) (-13.0638, -6.7278) (-13.0595, -6.7264) (-13.0552, -6.7249) (-13.0511, -6.7235) (-13.0469, -6.7221) (-13.0429, -6.7207) (-13.0388, -6.7193) (-13.0349, -6.7179) (-13.0309, -6.7165) (-13.0271, -6.7152) (-13.0232, -6.7138) (-13.0195, -6.7125) (-13.0158, -6.7111) (-13.0121, -6.7098) (-13.0085, -6.7085) (-13.005, -6.7072) (-13.0015, -6.7059) (-12.998, -6.7046) (-12.9946, -6.7033) (-12.9913, -6.7021) (-12.988, -6.7008) (-12.9848, -6.6996) (-12.9816, -6.6984) (-12.9785, -6.6972) (-12.9755, -6.696) (-12.9725, -6.6948) (-12.9695, -6.6937) (-12.9667, -6.6925) (-12.9638, -6.6914) (-12.9611, -6.6903) (-12.9584, -6.6892) (-12.9557, -6.6881) (-12.9531, -6.6871) (-12.9506, -6.686) (-12.9482, -6.685) (-12.9457, -6.684) (-12.9434, -6.683) (-12.9411, -6.6821) (-12.9389, -6.6811) (-12.9367, -6.6802) (-12.9346, -6.6793) (-12.9326, -6.6784) (-12.9306, -6.6775) (-12.9287, -6.6767) (-12.9269, -6.6759) (-12.9251, -6.6751) (-12.9234, -6.6743) (-12.9217, -6.6736) (-12.9201, -6.6729) (-12.9186, -6.6722) (-12.9171, -6.6715) (-12.9157, -6.6709) (-12.9144, -6.6703) (-12.9132, -6.6697) (-12.912, -6.6691) (-12.9108, -6.6686) (-12.9098, -6.6681) (-12.9088, -6.6676) (-12.9079, -6.6672) (-12.9071, -6.6668) (-12.9063, -6.6664) (-12.9056, -6.6661) (-12.905, -6.6658) (-12.9044, -6.6655) (-12.9039, -6.6652) (-12.9036, -6.6651) (-12.9034, -6.665) (-12.9033, -6.6649) (-12.9032, -6.6649) knots -1 -1 -1 -1 -1 -1 -0.99583333 -0.99166667 -0.9875 -0.98333333 -0.97916667 -0.975 -0.97083333 -0.96666667 -0.9625 -0.95833333 -0.95416667 -0.95 -0.94583333 -0.94166667 -0.9375 -0.93333333 -0.92916667 -0.925 -0.92083333 -0.91666667 -0.9125 -0.90833333 -0.90416667 -0.9 -0.89583333 -0.89166667 -0.8875 -0.88333333 -0.87916667 -0.875 -0.87083333 -0.86666667 -0.8625 -0.85833333 -0.85416667 -0.85 -0.84583333 -0.84166667 -0.8375 -0.83333333 -0.82916667 -0.825 -0.82083333 -0.81666667 -0.8125 -0.80833333 -0.80416667 -0.8 -0.79583333 -0.79166667 -0.7875 -0.78333333 -0.77916667 -0.775 -0.77083333 -0.76666667 -0.7625 -0.75833333 -0.75416667 -0.75 -0.74583333 -0.74166667 -0.7375 -0.73333333 -0.72916667 -0.725 -0.72083333 -0.71666667 -0.7125 -0.70833333 -0.70416667 -0.7 -0.69583333 -0.69166667 -0.6875 -0.68333333 -0.67916667 -0.675 -0.67083333 -0.66666667 -0.6625 -0.65833333 -0.65416667 -0.65 -0.64583333 -0.64166667 -0.6375 -0.63333333 -0.62916667 -0.625 -0.62083333 -0.61666667 -0.6125 -0.60833333 -0.60416667 -0.6 -0.59583333 -0.59166667 -0.5875 -0.58333333 -0.57916667 -0.575 -0.57083333 -0.56666667 -0.5625 -0.55833333 -0.55416667 -0.55 -0.54583333 -0.54166667 -0.5375 -0.53333333 -0.52916667 -0.525 -0.52083333 -0.51666667 -0.5125 -0.50833333 -0.50416667 -0.5 -0.49583333 -0.49166667 -0.4875 -0.48333333 -0.47916667 -0.475 -0.47083333 -0.46666667 -0.4625 -0.45833333 -0.45416667 -0.45 -0.44583333 -0.44166667 -0.4375 -0.43333333 -0.42916667 -0.425 -0.42083333 -0.41666667 -0.4125 -0.40833333 -0.40416667 -0.4 -0.39583333 -0.39166667 -0.3875 -0.38333333 -0.37916667 -0.375 -0.37083333 -0.36666667 -0.3625 -0.35833333 -0.35416667 -0.35 -0.34583333 -0.34166667 -0.3375 -0.33333333 -0.32916667 -0.325 -0.32083333 -0.31666667 -0.3125 -0.30833333 -0.30416667 -0.3 -0.29583333 -0.29166667 -0.2875 -0.28333333 -0.27916667 -0.275 -0.27083333 -0.26666667 -0.2625 -0.25833333 -0.25416667 -0.25 -0.24583333 -0.24166667 -0.2375 -0.23333333 -0.22916667 -0.225 -0.22083333 -0.21666667 -0.2125 -0.20833333 -0.20416667 -0.2 -0.19583333 -0.19166667 -0.1875 -0.18333333 -0.17916667 -0.175 -0.17083333 -0.16666667 -0.1625 -0.15833333 -0.15416667 -0.15 -0.14583333 -0.14166667 -0.1375 -0.13333333 -0.12916667 -0.125 -0.12083333 -0.11666667 -0.1125 -0.10833333 -0.10416667 -0.1 -0.09583333 -0.09166667 -0.0875 -0.08333333 -0.07916667 -0.075 -0.07083333 -0.06666667 -0.0625 -0.05833333 -0.05416667 -0.05 -0.04583333 -0.04166667 -0.0375 -0.03333333 -0.02916667 -0.025 -0.02083333 -0.01666667 -0.0125 -0.00833333 -0.00416667 0 0 0 0 0 0
  line L10 (-12.9032, -6.6649) -> (-12.9026, -6.6646)
  line L11 (-12.9026, -6.6646) -> (-12.2165, -6.3102)
  arc A14 (-12.2165, -6.3102) -> (-11.5731, -7.4247) centre (0, 0) ccw
  line L12 (-11.5731, -7.4247) -> (-12.223, -7.8417)
  line L13 (-12.223, -7.8417) -> (-12.2236, -7.8421)